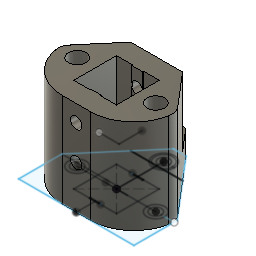
Bottom Tower support heavy duty R2 v5 (Autodesk Fusion 360 design; units mm, degrees)
Autodesk Fusion 360 part; units mm, degrees
note: some values were not read from the file. Chosen so that the rebuilt part matches the saved one: which face or edge a step refers to. Set by a fixed rule: which sketch regions a step uses.
sketch "Sketch1" plane through (0, 0, 0) normal (0, 1, 0) x (1, 0, 0)
  line L0 (0, 0) -> (18.8, 0)
  line L1 (0, 0) -> (-18.8, 0)
  line L2 (0, 0) -> (0, 22.6)
  circle A0 centre (18.8, 0) radius 2.625
  circle A1 centre (-18.8, 0) radius 2.625
  circle A2 centre (18.8, 0) radius 4.2
  circle A3 centre (-18.8, 0) radius 4.2
  line L3 (10.215, -10.215) -> (-10.215, -10.215)
  line L4 (-10.215, -10.215) -> (-10.215, 10.215)
  line L5 (-10.215, 10.215) -> (10.215, 10.215)
  line L6 (10.215, 10.215) -> (10.215, -10.215)
  line L7 (10.215, -10.215) -> (-10.215, 10.215) construction
  line L8 (-10.215, -10.215) -> (10.215, 10.215) construction
  circle A4 centre (0, 22.6) radius 2.55
  line L9 (0, 10.215) -> (2.6, 10.215)
  line L10 (0, 10.215) -> (-2.6, 10.215)
  line L11 (0, -10.215) -> (2.6, -10.215)
  line L12 (0, -10.215) -> (-2.6, -10.215)
  line L13 (-2.6, -10.215) -> (2.6, -10.215)
  line L14 (2.6, -10.215) -> (2.6, -9.765)
  line L15 (2.6, -9.765) -> (-2.6, -9.765)
  line L16 (-2.6, -9.765) -> (-2.6, -10.215)
  line L17 (2.6, 10.215) -> (-2.6, 10.215)
  line L18 (-2.6, 10.215) -> (-2.6, 9.765)
  line L19 (-2.6, 9.765) -> (2.6, 9.765)
  line L20 (2.6, 9.765) -> (2.6, 10.215)
  circle A5 centre (0, 22.6) radius 5
  line L21 (0, -10.215) -> (0, -19.215)
  line L22 (0, 10.215) -> (0, 19.215)
  line L23 (0, 0) -> (5.2, 0)
  line L24 (-5.2, 0) -> (5.2, 0) construction
  line L25 (23, 0) -> (27.55, 0)
  line L26 (27.55, -19.215) -> (-27.55, -19.215)
  line L27 (-27.55, -19.215) -> (-27.55, 1.415)
  line L28 (27.55, 1.415) -> (27.55, -19.215)
  line L29 (0, 19.215) -> (12.3767, 19.215)
  line L30 (0, 19.215) -> (-12.3767, 19.215)
  line L31 (-12.3767, 19.215) -> (12.3767, 19.215)
  line L32 (3, 30.215) -> (-3, 30.215)
  line L33 (-18, 30.215) -> (-18, 19.215)
  line L34 (0, 30.215) -> (-3, 30.215)
  line L35 (0, 10.215) -> (0, 1.415)
  line L36 (0, 1.415) -> (-27.55, 1.415)
  line L37 (-27.55, 1.415) -> (-3, 30.215)
  line L38 (-27.55, 19.215) -> (-18, 19.215)
  line L39 (-12.3767, 19.215) -> (12.3767, 19.215)
  line L40 (27.55, 1.415) -> (3, 30.215)
  circle A6 centre (0, 22.6) radius 4.2
  dimension "d1" = 18.8
  dimension "d2" = 18.8
  dimension "d3" = 22.6
  dimension "d4" = 5.25
  dimension "d5" = 5.25
  dimension "d6" = 8.4
  dimension "d7" = 8.4
  dimension "d8" = 20.43
  dimension "d9" = 20.43
  dimension "d10" = 5.1
  dimension "d11" = 2.6
  dimension "d12" = 2.6
  dimension "d13" = 2.6
  dimension "d14" = 2.6
  dimension "d15" = 0.45
  dimension "d16" = 0.45
  dimension "d17" = 10
  dimension "d18" = 9
  dimension "d19" = 9
  dimension "d20" = 5.2
  dimension "d21" = 4.55
  dimension "d23" = 18
  dimension "d25" = 11
  dimension "d26" = 3
  dimension "d27" = 8.8
  dimension "d30" = 8.4
  constraint coincident L0.start L1.start
  constraint horizontal L0
  constraint parallel L0 L1
  constraint perpendicular L0 L2
  constraint coincident L0.end A0.centre
  constraint coincident L1.end A1.centre
  constraint concentric A1 A3
  constraint horizontal L3
  constraint perpendicular L3 L4
  constraint parallel L3 L5
  constraint parallel L4 L6
  constraint coincident L7 L0.start
  constraint coincident L8 L0.start
  constraint coincident L2.end A4.centre
  constraint midpoint L5 L9.start
  constraint perpendicular L2 L9
  constraint perpendicular L2 L10
  constraint midpoint L3 L11.start
  constraint parallel L3 L11
  constraint parallel L3 L12
  constraint horizontal L13
  constraint vertical L14
  constraint horizontal L15
  constraint vertical L16
  constraint horizontal L17
  constraint vertical L18
  constraint horizontal L19
  constraint vertical L20
  constraint concentric A4 A5
  constraint perpendicular L12 L21
  constraint perpendicular L10 L22
  constraint perpendicular L2 L23
  constraint coincident L23.end L24.end
  constraint parallel L0 L24
  constraint midpoint L24 L0.start
  constraint coincident A2 L25.start
  constraint horizontal L25
  constraint horizontal L26
  constraint perpendicular L26 L27
  constraint parallel L26 L38
  constraint parallel L27 L28
  constraint perpendicular L22 L29
  constraint perpendicular L22 L30
  constraint horizontal L31
  constraint horizontal L32
  constraint vertical L33
  constraint parallel L32 L34
  constraint perpendicular L10 L35
  constraint perpendicular L27 L36
  constraint coincident L32 L34.start
  constraint coincident L37 L30.end
  constraint collinear L38 L39
  constraint symmetric L2 L32.end L32.start
  constraint symmetric L2 L27.end L28.start
  constraint coincident L40 L29.end
  measures "d1" distance of L0.start L0.end
  measures "d2" distance of L0.start L1.end
  measures "d3" distance of L0.start L2.end
  measures "d4" diameter of A0
  measures "d5" diameter of A1
  measures "d6" diameter of A2
  measures "d7" diameter of A3
  measures "d8" distance of L4.end L5.end
  measures "d9" distance of L3.end L4.end
  measures "d10" diameter of A4
  measures "d11" distance of L9.start L9.end
  measures "d12" distance of L9.start L10.end
  measures "d13" distance of L11.start L11.end
  measures "d14" distance of L11.start L12.end
  measures "d15" distance of L12.end L15.end
  measures "d16" distance of L9.end L19.end
  measures "d17" diameter of A5
  measures "d18" distance of L11.start L21.end
  measures "d19" distance of L9.start L22.end
  measures "d20" distance of L0.start L23.end
  measures "d21" distance of L25.start L25.end
  measures "d23" distance of L22.end L33.end
  measures "d25" distance of L33.end L33.start
  measures "d26" distance of L34.start L32.end
  measures "d27" distance of L9.start L35.end
  measures "d30" diameter of A6
extrude "Extrude1" add sketch "Sketch1" along normal blind 45 contours L1 A3 L3 L4 L12 L13 L21 L26 L27 L36 | L1 A3 L4 L36 | L0 L2 A2 L5 L6 L9 L17 A5 L22 L25 L28 L29 L31 L39 L40 | L0 A2 L3 L6 L11 L13 L21 L25 L26 L28 | L2 A3 L4 L5 L10 L17 A5 L22 L30 L31 L36 L37 L39 | L2 L5 L10 L17 L18 L19 L35 | L2 L5 L9 L17 L19 L20 L35 | L3 L11 L12 L13 L14 L15 L16 | L2 A5 L22 L30 L31 L39 A6 | L2 A5 L22 L29 L31 L39 A6 | L2 L22 L30 L31 L39 A6 | L2 L22 L29 L31 L39 A6
extrude "Extrude2" add sketch "Sketch1" along normal blind 12 contours A5 L29 L30 L31 L32 L34 L37 L39 L40 | A5 L29 L30 L31 L39 A6 | L29 L30 L31 L39 A6
extrude "Extrude3" cut sketch "Sketch1" along normal blind 2.8 contours L2 A5 L22 L30 L31 L39 A6 | L2 A5 L22 L29 L31 L39 A6 | L2 L22 L30 L31 L39 A6 | L2 L22 L29 L31 L39 A6 | A5 L29 L30 L31 L39 A6 | L29 L30 L31 L39 A6
hole "Hole1" at (0, 12, -22.6) direction (0, -1, 0) diameter 8.3 depth 4.5 tip angle 180
sketch "Sketch2" plane through (0, 0, -19.215) normal (0, 0, -1) x (-1, 0, 0)
  line L0 (-12.3767, 12) -> (-2.4009, 12)
  line L1 (-2.4009, 12) -> (2.4009, 12)
  line L2 (2.4009, 12) -> (12.3767, 12)
  line L3 (12.3767, 12) -> (12.3767, 45)
  line L4 (12.3767, 45) -> (-12.3767, 45)
  line L5 (-12.3767, 45) -> (-12.3767, 12)
  line L6 (0, 45) -> (0, 12)
  line L7 (0, 12) -> (0, 20.6)
  circle A0 centre (0, 20.6) radius 7.65
  line L8 (0, 45) -> (0, 37)
  circle A1 centre (0, 37) radius 7.65
  circle A2 centre (0, 20.6) radius 2.725
  circle A3 centre (0, 37) radius 2.725
  dimension "d40" = 8.6
  dimension "d41" = 15.3
  dimension "d42" = 8
  dimension "d43" = 15.3
  dimension "d44" = 5.45
  dimension "d45" = 5.45
  constraint midpoint L4 L6.start
  constraint midpoint L1 L6.end
  constraint coincident L6 L7.end
  constraint perpendicular L1 L7
  constraint coincident L7.end A0.centre
  constraint perpendicular L4 L8
  constraint coincident L8.end A1.centre
  measures "d40" distance of L6.end L7.end
  measures "d41" diameter of A0
  measures "d42" distance of L6.start L8.end
  measures "d43" diameter of A1
  measures "d44" diameter of A2
  measures "d45" diameter of A3
extrude "Extrude4" cut sketch "Sketch2" against normal blind 56 contours L6 L7 A2 | L6 L7 A2 | L6 L8 A3 | L6 L8 A3
extrude "Extrude5" add sketch "Sketch1" along normal blind 36 contours L1 A1 A3 L36 | L1 A1 A3 L36 | A2 | A1 A3 L36
fillet "Fillet2" radius 21 2 edges at (-27.55, 22.5, 19.215) (27.55, 22.5, 19.215)
fillet "Fillet3" radius 7 2 edges at (-27.5468, 22.5, -1.4187) (27.5468, 22.5, -1.4187)
fillet "Fillet4" radius 5 2 edges at (3, 6, -30.215) (-3, 6, -30.215)
chamfer "Chamfer1" distance 0.3 distance2 1 1 edges at (-4.6616, 2.8, -20.7919) measured on face at (4.9752, 0.9333, -22.1022)
chamfer "Chamfer2" distance 0.23 distance2 0.2 10 edges at (16.3526, 0, -0.9492) (10.215, 0, 0) (6.4075, 0, -10.215) (-6.4075, 0, -10.215) (-10.215, 0, 0) (0, 0, -9.765) (-21.2474, 0, -0.9492) (-6.4075, 0, 10.215) (0, 0, 9.765) (6.4075, 0, 10.215) measured on face at (21.4217, 24, 0.1308) measured on face at (10.215, 30, 3.405) measured on face at (7.7167, 21.9219, -10.215) measured on face at (-7.7183, 21.8667, -10.215) measured on face at (-10.215, 30, -3.405) measured on face at (-0.0676, 5.9609, -9.765) measured on face at (-16.1783, 24, 0.1308) measured on face at (-7.7183, 21.8667, 10.215) measured on face at (0.0676, 5.9609, 9.765) measured on face at (7.7167, 21.9219, 10.215)
named bodies: "Bottom Tower support heavy duty R2"
